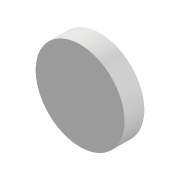
# Autodesk Inventor part: MATERIAL MOLDE 1
Saved by Autodesk Inventor 2021.4 (Build 254397000, 397)
## iProperties
Created: 2023-02-13
Part Number: MATERIAL MOLDE 1
Material: Generic
Document SubType Name: Modeling
Designer: rodar
Density: 1 g/cm^3
Appearance: Default
Author: rodar
Autodesk Inventor part; units mm, degrees
sketch "Sketch1" plane through (0, 0, 0) normal (0, 0, 1) x (1, 0, 0)
  circle A0 centre (38.1, 38.1) radius 36
  point P0 (0, 0)
  dimension "d0" = 38.1
  dimension "d1" = 38.1
  dimension "d2" = 72
  constraints: 1 centre point
  measures "d0" horizontal distance of A0.centre point (0, 0)
  measures "d1" horizontal distance of point (0, 0) A0.centre
  measures "d2" diameter of A0
ref_plane "Work Plane1" through (-3.81, -3.81, -16.05) normal (0, 0, 1) x (1, 0, 0)
ref_plane "Work Plane2" through (-3.81, -3.81, -15.05) normal (0, 0, 1) x (1, 0, 0)
ref_plane "Work Plane3" through (-3.81, -3.81, -16.05) normal (0, 0, 1) x (1, 0, 0)
extrude "Extrusion1" add sketch "Sketch1" against normal up to surface (16.05 mm away)
body "Solid1"
